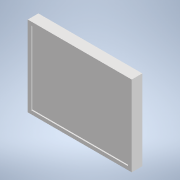
# Autodesk Inventor part: Monitor
Saved by Autodesk Inventor 2022 (Build 260153000, 153)
## iProperties
Created: 2023-12-20
Part Number: Monitor
Material: Generic
Document SubType Name: Modeling
Designer: Petr Černý
Density: 1 g/cm^3
Appearance: Default
Author: Petr Černý
Autodesk Inventor part; units mm, degrees
ref_plane "YZ Plane" through (0, 0, 0) normal (1, 0, 0) x (0, 1, 0)
ref_plane "XZ Plane" through (0, 0, 0) normal (0, 1, 0) x (-1, 0, 0)
ref_plane "XY Plane" through (0, 0, 0) normal (0, 0, 1) x (1, 0, 0)
sketch "Sketch1" plane through (0, 0, 0) normal (0, 0, 1) x (1, 0, 0)
  line L0 (90.3787, -90.3787) -> (-349.6213, -90.3787)
  line L1 (-349.6213, -90.3787) -> (-349.6213, -430.3787)
  line L2 (-349.6213, -430.3787) -> (90.3787, -430.3787)
  line L3 (90.3787, -430.3787) -> (90.3787, -90.3787)
  point P0 (0, 0)
  dimension "d0" = 440
  dimension "d1" = 340
  constraints: 8 end point, 2 parallel, 1 horizontal, 1 perpendicular
  measures "d0" distance of L2.end L1.end
  measures "d1" distance of L1.end L0.end
extrude "Extrusion1" add sketch "Sketch1" along normal blind 45
sketch "Sketch2" plane through (0, 0, 45) normal (0, 0, 1) x (1, 0, 0)
  line L0 (-334.6213, -105.3787) -> (75.3787, -105.3787)
  line L1 (75.3787, -105.3787) -> (75.3787, -415.3787)
  line L2 (75.3787, -415.3787) -> (-334.6213, -415.3787)
  line L3 (-334.6213, -415.3787) -> (-334.6213, -105.3787)
  line L4 (90.3787, -430.3787) -> (90.3787, -90.3787) projected
  line L5 (90.3787, -90.3787) -> (-349.6213, -90.3787) projected
  point P0 (0, 0)
  dimension "d4" = 410
  dimension "d5" = 310
  dimension "d6" = 15
  dimension "d7" = 15
  constraints: 8 end point, 2 parallel, 1 horizontal, 1 perpendicular
  measures "d4" distance of L0.start L0.end
  measures "d5" distance of L0.end L1.end
  measures "d6" distance between parallel lines of L4 L1
  measures "d7" distance between parallel lines of L5 L0
extrude "Extrusion2" cut sketch "Sketch2" against normal blind 5
sketch "Sketch3" plane through (0, 0, 0) normal (0, 0, -1) x (-1, 0, 0)
  line L0 (-35.3787, -145.3787) -> (294.6213, -145.3787)
  line L1 (294.6213, -145.3787) -> (294.6213, -375.3787)
  line L2 (294.6213, -375.3787) -> (-35.3787, -375.3787)
  line L3 (-35.3787, -375.3787) -> (-35.3787, -145.3787)
  line L4 (349.6213, -430.3787) -> (-90.3787, -430.3787) projected
  line L5 (-90.3787, -430.3787) -> (-90.3787, -90.3787) projected
  point P0 (0, 0)
  dimension "d10" = 330
  dimension "d11" = 230
  dimension "d12" = 55
  dimension "d13" = 55
  constraints: 8 end point, 2 parallel, 1 horizontal, 1 perpendicular
  measures "d10" distance of L1.end L2.end
  measures "d11" distance of L0.end L1.end
  measures "d12" distance between parallel lines of L4 L2
  measures "d13" distance between parallel lines of L5 L3
extrude "Extrusion3" add sketch "Sketch3" along normal blind 42
body "Solid1"
